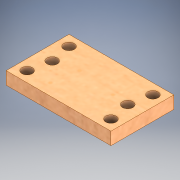
# Autodesk Inventor part: hold_motor_bottom
Saved by Autodesk Inventor 2020 (Build 240168000, 168)
## iProperties
Created: 2019-12-02
Part Number: hold_motor_bottom
Material: Bois (cerisier)
Document SubType Name: Modeling
Designer: bapti
Density: 0.63 g/cm^3
Appearance: Cerisier - Faible lustre naturel
Author: bapti
Autodesk Inventor part; units mm, degrees
ref_plane "YZ Plane" through (0, 0, 0) normal (1, 0, 0) x (0, 1, 0)
ref_plane "XZ Plane" through (0, 0, 0) normal (0, 1, 0) x (-1, 0, 0)
ref_plane "XY Plane" through (0, 0, 0) normal (0, 0, 1) x (1, 0, 0)
sketch "Esquisse1" plane through (0, 0, 0) normal (0, 1, 0) x (-1, 0, 0)
  line L0 (0, 0) -> (50, 0)
  line L1 (50, 0) -> (50, -30)
  line L2 (50, -30) -> (0, -30)
  line L3 (0, -30) -> (0, 0)
  line L4 (50, -15) -> (0, -15) construction
  line L5 (50, -10) -> (0, -10) construction
  line L6 (50, -20) -> (0, -20) construction
  circle A0 centre (45, -5) radius 2.5
  line L7 (25, 0) -> (25, -30) construction
  circle A1 centre (5, -5) radius 2.5
  circle A2 centre (45, -25) radius 2.5
  circle A3 centre (5, -25) radius 2.5
  circle A4 centre (43, -15) radius 2.5
  circle A5 centre (7, -15) radius 2.5
  dimension "d0" = 50
  dimension "d2" = 10
  dimension "d3" = 10
  dimension "d4" = 5
  dimension "d10" = 5
  dimension "d11" = 18
  dimension "d12" = 5
  dimension "d13" = 10
  dimension "d14" = 20
  constraints: 16 end point, 6 centre point, 5 point on line, 4 midpoint, 4 symmetric about line, 3 perpendicular, 2 parallel, 1 horizontal, 4 other
  measures "d0" distance of L0.start L0.end
  measures "d2" distance between parallel lines of L5 L0
  measures "d3" distance of L1.end L6.start
  measures "d4" diameter of A0
  measures "d10" diameter of A4
  measures "d11" distance from line of L7 A4.centre
  measures "d12" distance from line of L5 A0.centre
  measures "d13" distance of L6.start L5.start
  measures "d14" distance from line of L7 A0.centre
extrude "Extrusion1" add sketch "Esquisse1" along normal blind 6
equation "\"d3\" = d2"
